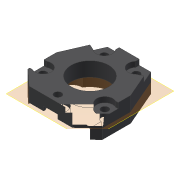
# Autodesk Inventor part: linact_thumb_front
Saved by Autodesk Inventor 2014 (Build 180170000, 170)
## iProperties
Created: 2015-05-22
Part Number: linact_thumb_front
Material: Generic
Document SubType Name: Modeling
Designer: Martin
Density: 1 g/cm^3
Appearance: Default
Author: Martin
Autodesk Inventor part; units mm, degrees
ref_plane "YZ Plane" through (0, 0, 0) normal (1, 0, 0) x (0, 1, 0)
ref_plane "XZ Plane" through (0, 0, 0) normal (0, 1, 0) x (-1, 0, 0)
ref_plane "Work Plane1" through (0, 0, 0) normal (0, 0, 1) x (1, 0, 0)
sketch "Sketch1" plane through (0, 0, 0) normal (0, 0, 1) x (1, 0, 0)
  line L0 (-6.075, -22) -> (6.075, -22) projected
  line L1 (-6.075, -22) -> (-10.3994, -18) projected
  line L2 (-10.3994, -18) -> (-10.3994, -10) projected
  line L3 (-10.3994, -10) -> (-6.075, 0) projected
  line L4 (6.075, 0) -> (-6.075, 0) projected
  line L5 (6.075, 0) -> (10.3994, -10) projected
  line L6 (10.3994, -10) -> (10.3994, -18) projected
  line L7 (10.3994, -18) -> (6.075, -22) projected
  circle A0 centre (0, -11) radius 3.4 projected
  circle A1 centre (0, -20) radius 1 projected
  circle A2 centre (8.6494, -15.5) radius 1 projected
  circle A3 centre (-8.6494, -15.5) radius 1 projected
  circle A4 centre (0, -20) radius 2.5
  line L8 (-2, -21.5) -> (-2, -22)
  line L9 (2, -21.5) -> (2, -22)
  line L10 (0, -20) -> (0, -22) construction
  circle A5 centre (0, -11) radius 5.25
  line L11 (0, 4.5) -> (0, -27) projected
  circle A6 centre (-5, -2.5) radius 1 projected
  circle A7 centre (5, -2.5) radius 1 projected
  point P0 (0, 0)
  dimension "d0" = 5
  dimension "d1" = 4
  dimension "d2" = 10.5
  constraints: 6 end point, 2 centre point, 2 coincident, 2 point on circle, 2 point on line, 1 midpoint, 1 parallel, 1 perpendicular, 1 other
  measures "d0" diameter of A4
  measures "d1" distance between parallel lines of L9 L8
  measures "d2" diameter of A5
extrude "ext_main" add sketch "Sketch1" along normal blind 4 contours L1 L2 L3 L4 L11 A5 A4 L8 L0 | L8 A4 L0 | A4 L11 A1 L0 | L11 A1 A4 L0 | L11 A5 L4 L5 L6 L7 L0 L9 A4 | A4 L9 L0
sketch "Sketch2" plane through (0, 0, 0) normal (0, 0, -1) x (-1, 0, 0)
  circle A0 centre (0, -20) radius 2.5 projected
  line L0 (-2, -21.5) -> (-2, -22) projected
  line L1 (2, -21.5) -> (2, -22) projected
  line L2 (-2, -22) -> (2, -22)
  constraints: 2 end point, 1 perpendicular
extrude "ext_cut_gearhousing" cut sketch "Sketch2" against normal blind 1.2
sketch "Sketch3" plane through (0, 0, 0) normal (0, 0, 1) x (1, 0, 0)
  line L0 (-10.3994, -18) -> (-10.3994, -10) projected
  line L1 (-6.075, -22) -> (-10.3994, -18) projected
  line L2 (-6.075, -22) -> (6.075, -22) projected
  line L3 (10.3994, -18) -> (6.075, -22) projected
  line L4 (10.3994, -10) -> (10.3994, -18) projected
  line L5 (6.075, 0) -> (10.3994, -10) projected
  line L6 (6.075, 0) -> (-6.075, 0) projected
  line L7 (-10.3994, -10) -> (-6.075, 0) projected
  circle A0 centre (-8.6494, -15.5) radius 1 projected
  circle A1 centre (8.6494, -15.5) radius 1 projected
  circle A2 centre (0, -20) radius 1 projected
  circle A3 centre (0, -11) radius 3.4 projected
  circle A4 centre (0, -20) radius 8 construction
  circle A5 centre (5.075, -11) radius 1 projected
  circle A6 centre (-5.075, -11) radius 1 projected
  circle A7 centre (-5.075, -11) radius 3 construction
  circle A8 centre (5.075, -11) radius 3 construction
  line L8 (-8.6494, -16.5) -> (-8.6494, -19.6187)
  line L9 (-5.075, -11) -> (-8.6494, -15.5) construction
  line L10 (5.075, -11) -> (8.6494, -15.5) construction
  line L11 (8.6494, -15.5) -> (8.6494, -19.6187) construction
  line L12 (8.6494, -16.5) -> (8.6494, -19.6187)
  arc A9 (-8.0274, -14.717) -> (-8.6494, -16.5) centre (-8.6494, -15.5) ccw
  arc A10 (8.6494, -16.5) -> (8.0274, -14.717) centre (8.6494, -15.5) ccw
  line L13 (-8.6494, -19.6187) -> (-10.3994, -18)
  line L14 (10.3994, -18) -> (8.6494, -19.6187)
  circle A11 centre (0, -11) radius 8.25 construction
  line L15 (-7.6085, -14.1895) -> (-8.0274, -14.717)
  line L16 (8.0274, -14.717) -> (7.6085, -14.1895)
  circle A12 centre (-5, -2.5) radius 1 projected
  circle A13 centre (5, -2.5) radius 1 projected
  arc A14 (7.6085, -14.1895) -> (-7.6085, -14.1895) centre (0, -11) ccw
  point P0 (-6.9409, -13.3491)
  point P1 (5.075, -8)
  point P2 (-5.075, -8)
  point P3 (6.9409, -13.3491)
  dimension "d7" = 16
  dimension "d8" = 6
  dimension "d20" = 16.5
  constraints: 18 end point, 16 point on circle, 10 point on line, 7 centre point, 4 coincident, 4 equal radius, 3 collinear, 1 perpendicular
  measures "d7" diameter of A4
  measures "d8" diameter of A7
  measures "d20" diameter of A11
ref_plane "Work Plane2" through (-10.3994, -22, -2.8) normal (0, 0, 1) x (1, 0, 0)
extrude "ext_base" add sketch "Sketch3" against normal up to surface (2.8 mm away) contours L0 L7 L6 L5 L4 L3 L12 A1 L16 A14 L15 A0 L8 L1
sketch "Sketch4" plane through (0, 0, 4) normal (0, 0, 1) x (1, 0, 0)
  circle A0 centre (8.6494, -15.5) radius 1 projected
  circle A1 centre (-8.6494, -15.5) radius 1 projected
  line L0 (10.3994, -18) -> (10.3994, -10) projected
  line L1 (-10.3994, -10) -> (-10.3994, -18) projected
  circle A2 centre (-8.6494, -15.5) radius 2.25
  circle A3 centre (8.6494, -15.5) radius 2.25
  line L2 (-9.6802, -13.5) -> (-10.3994, -13.5)
  line L3 (-9.6802, -17.5) -> (-10.3994, -17.5)
  line L4 (-8.6494, -15.5) -> (-10.3994, -15.5) construction
  line L5 (8.6494, -15.5) -> (10.3994, -15.5)
  line L6 (9.6802, -13.5) -> (10.3994, -13.5)
  line L7 (9.6802, -17.5) -> (10.3994, -17.5)
  circle A4 centre (-5, -2.5) radius 1 projected
  circle A5 centre (5, -2.5) radius 1 projected
  line L8 (10.3994, -10) -> (6.075, 0) projected
  line L9 (6.075, 0) -> (-6.075, 0) projected
  line L10 (-6.075, 0) -> (-10.3994, -10) projected
  circle A6 centre (-5, -2.5) radius 2.25
  circle A7 centre (5, -2.5) radius 2.25
  line L11 (-2.825, -1.9239) -> (-2.825, 0)
  line L12 (-6.8699, -3.7514) -> (-7.5669, -3.45)
  line L13 (0, 4.4) -> (0, -26.4) projected
  line L14 (2.825, -1.9239) -> (2.825, 0)
  line L15 (6.8699, -3.7514) -> (7.5669, -3.45)
  point P0 (0, 0)
  dimension "d11" = 4.5
  dimension "d12" = 4
  dimension "d13" = 4
  dimension "d18" = 3.25
  dimension "d19" = 3.45
  constraints: 20 end point, 10 point on line, 8 perpendicular, 8 point on circle, 4 centre point, 4 coincident, 3 equal radius, 2 symmetric about line, 1 parallel, 4 other
  measures "d11" diameter of A2
  measures "d12" distance of L7.end L6.end
  measures "d13" distance of L3.end L2.end
  measures "d18" distance of L11.end L9.end
  measures "d19" vertical distance of L9.end L12.end
extrude "ext_cut_screwheads" cut sketch "Sketch4" against normal blind 1.5 contours L0 A3 | L2 A2 L1 | L11 A6 L10 L9 | L15 A7 L8 | L0 L7 A3 | A3 L6 L0 | A7 L8 | L8 A7 | A7 L14 L9 L8 | A6 L10 | L10 A6 | A6 L12 L10 | A2 L1 | A2 L3 L1 | A4 | A5 picked at (10.1112, -14.8737) picked at (-10.1494, -15.5)
equation "\"d11\" = screw_m2_head_maxsize"
equation "\"screw_m2_head_maxsize\" = 4.5"
body "Solid1"
